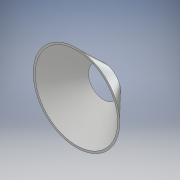
# Autodesk Inventor part: DPLX_P009_Wire_Mesh_reducer_Trans
Saved by Autodesk Inventor 2018 (Build 220112000, 112)
## iProperties
Created: 2018-06-07
Part Number: DPLX_P009_Wire_Mesh_reducer_Trans
Material: Generic
Document SubType Name: Modeling
Designer: DPLXuser
Density: 1 g/cm^3
Appearance: Default
Author: DPLXuser
Autodesk Inventor part; units mm, degrees
ref_plane "YZ Plane" through (0, 0, 0) normal (1, 0, 0) x (0, 1, 0)
ref_plane "XY Plane" through (0, 0, 0) normal (0, 0, 1) x (1, 0, 0)
sketch "Sketch1" plane through (0, 0, 0) normal (0, 1, 0) x (-1, 0, 0)
  circle A0 centre (0, 0) radius 15.9385
  dimension "d0" = 31.877
  constraints: 1 centre point, 1 coincident
  measures "d0" diameter of A0
ref_plane "Work Plane1" through (0, 10, 0) normal (0, 1, 0) x (-1, 0, 0)
sketch "Sketch7" plane through (0, 10, 0) normal (0, 1, 0) x (-1, 0, 0)
  circle A0 centre (0, 0) radius 6.35
  dimension "d16" = 12.7
  constraints: 1 centre point, 1 coincident
  measures "d16" diameter of A0
loft "Loft3" add profiles "Sketch1", "Sketch7"
shell "Shell3" thickness 0.533 removed faces 2 at (1.8127, 10, -0.4771) at (0.7499, 0, -4.3724)
sketch "Sketch8" plane through (0, 10, 0) normal (0, 1, 0) x (-1, 0, 0)
  circle A0 centre (0, 0) radius 6.35 projected
  constraints: 1 coincident
body "Solid3"
